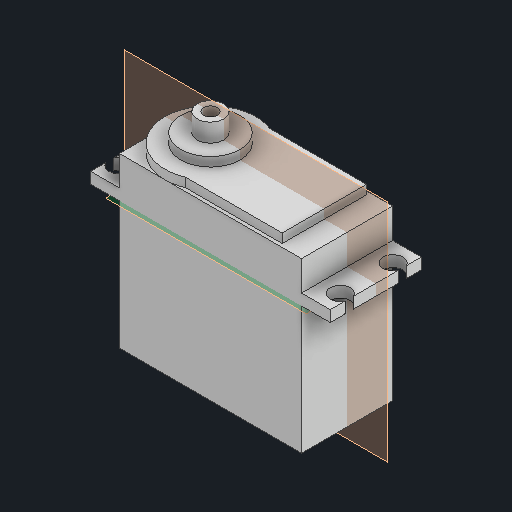
# Autodesk Inventor part: MG996R
Saved by Autodesk Inventor 2024 (Build 280153000, 153)
## iProperties
Created: 2025-09-12
Part Number: MG996R
Material: Generic
Document SubType Name: Modeling
Designer: kevin
Density: 1 g/cm^3
Appearance: Default
Author: kevin
Autodesk Inventor part; units mm, degrees
ref_plane "YZ Plane" through (0, 0, 0) normal (1, 0, 0) x (0, 1, 0)
ref_plane "XZ Plane" through (0, 0, 0) normal (0, 1, 0) x (-1, 0, 0)
sketch "Sketch1" plane through (0, 0, 0) normal (0, 1, 0) x (-1, 0, 0)
  line L0 (-20, 10) -> (20, 10)
  line L1 (20, 10) -> (20, -10)
  line L2 (20, -10) -> (-20, -10)
  line L3 (-20, -10) -> (-20, 10)
  line L4 (-20, 10) -> (20, -10) construction
  line L5 (20, 10) -> (-20, -10) construction
  point P0 (0, 0)
  dimension "d0" = 40
  dimension "d1" = 20
  constraints: 12 end point, 2 midpoint, 2 parallel, 1 horizontal, 1 perpendicular
  measures "d0" distance of L1.end L2.end
  measures "d1" distance of L0.end L1.end
extrude "Extrusion1" add sketch "Sketch1" along normal blind 37
sketch "Sketch2" plane through (0, 37, 0) normal (0, 1, 0) x (1, 0, 0)
  line L0 (20, 10) -> (-20, 10) projected
  line L1 (-20, 10) -> (-20, -10) projected
  line L2 (-20, -10) -> (20, -10) projected
  line L3 (20, -10) -> (20, 10) projected
  circle A0 centre (-10, 0) radius 10
  line L4 (-20, 10) -> (-20, -10) projected
  line L5 (15, -10) -> (15, 10)
  line L6 (15, 9.25) -> (-6.2003, 9.25)
  line L7 (-6.2003, -9.25) -> (15, -9.25)
  point P0 (0, 0)
  dimension "d4" = 5
  constraints: 6 end point, 4 point on line, 2 point on circle, 2 tangent, 1 centre point, 1 perpendicular
  measures "d4" distance between parallel lines of L3 L5
extrude "Extrusion2" add sketch "Sketch2" along normal blind 2 contours A0 | L5 L7 A0 L6
sketch "Sketch3" plane through (0, 39, 0) normal (0, 1, 0) x (1, 0, 0)
  line L0 (-6.2003, -9.25) -> (15, -9.25) projected
  line L1 (15, -9.25) -> (15, 9.25) projected
  line L2 (15, 9.25) -> (-6.2003, 9.25) projected
  arc A0 (-6.2003, 9.25) -> (-6.2003, -9.25) centre (-10, 0) ccw projected
  circle A1 centre (-10, 0) radius 6.5
  point P0 (0, 0)
  dimension "d8" = 13
  constraints: 1 centre point, 1 coincident
  measures "d8" diameter of A1
extrude "Extrusion3" add sketch "Sketch3" along normal blind 2 contours A1
sketch "Sketch4" plane through (-10, 41, 0) normal (0, 1, 0) x (1, 0, 0)
  circle A0 centre (0, 0) radius 6.5 projected
  circle A1 centre (0, 0) radius 2.9
  circle A2 centre (0, 0) radius 1.5
  point P0 (10, 0)
  dimension "d11" = 5.8
  dimension "d12" = 3
  constraints: 2 centre point, 2 coincident
  measures "d11" diameter of A1
  measures "d12" diameter of A2
extrude "Extrusion4" add sketch "Sketch4" along normal blind 4 contours A1
ref_plane "Work Plane1" through (0, 28, 0) normal (0, -1, 0) x (1, 0, 0)
sketch "Sketch5" plane through (0, 28, 0) normal (0, -1, 0) x (1, 0, 0)
  arc A0 (-10, -10) -> (-6.2003, -9.25) centre (-10, 0) ccw projected
  line L0 (-6.2003, -9.25) -> (15, -9.25) projected
  line L1 (15, -9.25) -> (15, 9.25) projected
  line L2 (15, 9.25) -> (-6.2003, 9.25) projected
  arc A1 (-6.2003, 9.25) -> (-10, 10) centre (-10, 0) ccw projected
  line L3 (-10, 10) -> (20, 10) projected
  line L4 (20, 10) -> (20, -10) projected
  line L5 (20, -10) -> (-10, -10) projected
  arc A2 (-10, 10) -> (-20, 0) centre (-10, 0) ccw projected
  line L6 (-20, 0) -> (-20, 10) projected
  line L7 (-20, 10) -> (-10, 10) projected
  arc A3 (-20, 0) -> (-10, -10) centre (-10, 0) ccw projected
  line L8 (-10, -10) -> (-20, -10) projected
  line L9 (-20, -10) -> (-20, 0) projected
  line L10 (-20, 10) -> (-26.3, 10)
  line L11 (-26.3, 10) -> (-26.3, -10)
  line L12 (-26.3, -10) -> (-20, -10)
  line L13 (-20, -10) -> (-20, 10)
  line L14 (20, 10) -> (26.3, 10)
  line L15 (26.3, 10) -> (26.3, -10)
  line L16 (26.3, -10) -> (20, -10)
  line L17 (20, -10) -> (20, 10)
  circle A4 centre (24.3, 5.8) radius 2.2
  line L18 (20, 5.8) -> (22.1, 5.8) construction
  line L19 (0, -10) -> (0, -15.1491)
  line L20 (20, 10) -> (20, -10) projected
  line L21 (20, 0) -> (22.5191, 0)
  line L22 (24.3, 8) -> (24.3, 10) construction
  circle A5 centre (24.3, -5.8) radius 2.2
  circle A6 centre (-24.3, 5.8) radius 2.2
  circle A7 centre (-24.3, -5.8) radius 2.2
  point P0 (0, 0)
  point P1 (26.3, -6.7165)
  point P2 (26.3, -4.8835)
  point P3 (26.3, 4.8835)
  point P4 (26.3, 6.7165)
  point P5 (-26.3, 6.7165)
  point P6 (-26.3, 4.8835)
  point P7 (-26.3, -4.8835)
  point P8 (-26.3, -6.7165)
  point P9 (-20, 0)
  dimension "d16" = 6.3
  dimension "d17" = 6.3
  dimension "d18" = 4.4
  dimension "d19" = 2.1
  dimension "d20" = 2
  constraints: 24 end point, 5 point on line, 4 centre point, 4 parallel, 4 perpendicular, 3 horizontal, 3 symmetric about line, 2 point on circle, 1 midpoint, 1 vertical, 3 other
  measures "d16" distance of L12.end L11.end
  measures "d17" distance of L15.end L16.end
  measures "d18" diameter of A4
  measures "d19" distance of L18.start L18.end
  measures "d20" distance of L22.start L22.end
extrude "Extrusion5" add sketch "Sketch5" against normal blind 2.45 contours L9 L12 L11 A7 A6 L10 L6 | L4 L14 L15 A4 A5 L16
equation "\"d16\" = d17"
body "Solid1"
